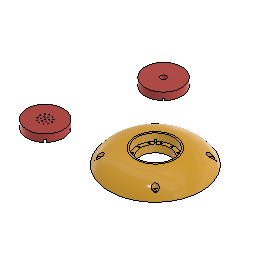
Chapeau (Autodesk Fusion 360 design; units mm, degrees)
Autodesk Fusion 360 part; units mm, degrees
note: some values were not read from the file. Set by a fixed rule: which sketch regions a step uses.
sketch "Sketch1" plane through (0, 0, 0) normal (0, 0, 1) x (1, 0, 0) in component "Chapeau"
  line L0 (-67.3, 67.3) -> (-82.7, 67.3)
  line L1 (-82.7, 67.3) -> (-82.7, 82.7)
  line L2 (-82.7, 82.7) -> (-67.3, 82.7)
  line L3 (-67.3, 82.7) -> (-67.3, 67.3)
  line L4 (-67.3, 67.3) -> (-82.7, 82.7) construction
  line L5 (-82.7, 67.3) -> (-67.3, 82.7) construction
  line L6 (0, 0) -> (0, 45.9001) construction
  line L7 (0, 0) -> (-36.9547, 0) construction
  line L8 (67.3, 82.7) -> (82.7, 82.7)
  line L9 (82.7, 82.7) -> (82.7, 67.3)
  line L10 (82.7, 67.3) -> (67.3, 67.3)
  line L11 (67.3, 67.3) -> (67.3, 82.7)
  line L12 (-82.7, -67.3) -> (-67.3, -67.3)
  line L13 (-67.3, -67.3) -> (-67.3, -82.7)
  line L14 (-67.3, -82.7) -> (-82.7, -82.7)
  line L15 (-82.7, -82.7) -> (-82.7, -67.3)
  line L16 (67.3, -67.3) -> (82.7, -67.3)
  line L17 (82.7, -67.3) -> (82.7, -82.7)
  line L18 (82.7, -82.7) -> (67.3, -82.7)
  line L19 (67.3, -82.7) -> (67.3, -67.3)
  circle A0 centre (0, 0) radius 125
  circle A1 centre (-75, 75) radius 3.1
  circle A2 centre (75, 75) radius 3.1
  circle A3 centre (-75, -75) radius 3.1
  circle A4 centre (75, -75) radius 3.1
  point P0 (-75, 75)
  dimension "d1" = 15.4
  dimension "d2" = 15.4
  dimension "d3" = 75
  dimension "d4" = 75
  dimension "d7" = 150
  dimension "d8" = -150
  dimension "d9" = 250
  dimension "d16" = 6.2
  dimension "d19" = 150
  dimension "d20" = -150
  constraint horizontal L0
  constraint perpendicular L0 L1
  constraint parallel L0 L2
  constraint parallel L1 L3
  constraint coincident L4 P0
  constraint coincident L5 P0
  constraint coincident L6.start L7.start
  constraint perpendicular L2 L6
  constraint perpendicular L6 L7
  constraint coincident P0 A1.centre
  measures "d1" distance of L1.end L2.end
  measures "d2" distance of L0.end L1.end
  measures "d3" vertical distance of L6.start A1.centre
  measures "d4" horizontal distance of L6.start A1.centre
  measures "d9" diameter of A0
  measures "d16" diameter of A1
extrude "Extrude1" add sketch "Sketch1" along normal blind 40 contours L0 L1 L2 L3 | L8 L9 L10 L11 | L12 L13 L14 L15 | L16 L17 L18 L19 | A0 | A1 | A2 | A3 | A4 makes body 1 in component "Chapeau"
fillet "Fillet1" radius 82.5 1 edges at (-116.5409, -45.2019, 40) on bodies 1 in component "Chapeau"
extrude "Extrude3" cut sketch "Sketch1" along normal blind 60 contours A1 | A2 | A3 | A4 bodies 1 in component "Chapeau"
extrude "Extrude2" cut sketch "Sketch1" along normal blind 10 contours L0 L1 L2 L3 | L8 L9 L10 L11 | L12 L13 L14 L15 | L16 L17 L18 L19 | A1 | A2 | A3 | A4 bodies 1 in component "Chapeau"
ref_plane "WorkPlane1" through (-75, 75, 14) normal (0, 0, -1) x (-1, 0, 0) in component "Chapeau"
sketch "Sketch2" plane through (75, -75, 14) normal (0, 0, -1) x (1, 0, 0) in component "Chapeau"
  circle A0 centre (-150, 0) radius 3.1
  circle A1 centre (-150, -150) radius 3.1
  circle A2 centre (0, -150) radius 3.1
  circle A3 centre (0, 0) radius 3.1
  circle A4 centre (-150, 0) radius 7.5
  circle A5 centre (-150, -150) radius 7.5
  circle A6 centre (0, -150) radius 7.5
  circle A7 centre (0, 0) radius 7.5
  dimension "d34" = 15
  dimension "d35" = 15
  dimension "d36" = 15
  dimension "d37" = 15
  constraint concentric A0 A4
  constraint concentric A1 A5
  constraint concentric A2 A6
  constraint concentric A3 A7
  measures "d34" diameter of A4
  measures "d35" diameter of A5
  measures "d36" diameter of A6
  measures "d37" diameter of A7
extrude "Extrude1'" cut sketch "Sketch2" against normal blind 55 bodies 1 in component "Chapeau"
sketch "Sketch4" plane through (0, 0, 40) normal (0, 0, 1) x (-1, 0, 0) in component "Chapeau"
  circle A0 centre (0, 0) radius 54.2893
  circle A1 centre (0, 0) radius 50
  circle A2 centre (0, 0) radius 40
  dimension "d53" = 100
  dimension "d54" = 10
  constraint concentric A0 A1
  constraint concentric A1 A2
  measures "d53" diameter of A1
  measures "d54" distance of A1 A2
extrude "Extrude3'" cut sketch "Sketch4" against normal through all contours A2 bodies 1 in component "Chapeau"
extrude "Extrude7" cut sketch "Sketch4" against normal blind 20 contours A1 bodies 1 in component "Chapeau"
sketch "Sketch1 (1)" plane through (0, 0, 20) normal (0, 0, 1) x (-1, 0, 0) in component "Chapeau"
  circle A0 centre (0, 0) radius 40
  circle A1 centre (0, 0) radius 54.2893
  circle A2 centre (0, -45) radius 2.5
  circle A3 centre (38.9711, -22.5) radius 2.5
  circle A4 centre (38.9711, 22.5) radius 2.5
  circle A5 centre (0, 45) radius 2.5
  circle A6 centre (-38.9711, 22.5) radius 2.5
  circle A7 centre (-38.9711, -22.5) radius 2.5
  circle A8 centre (0, -45) radius 1
  circle A9 centre (38.9711, -22.5) radius 1
  circle A10 centre (38.9711, 22.5) radius 1
  circle A11 centre (0, 45) radius 1
  circle A12 centre (-38.9711, 22.5) radius 1
  circle A13 centre (-38.9711, -22.5) radius 1
  circle A14 centre (0, 0) radius 40
  circle A15 centre (0, 0) radius 50
  line L0 (0, 0) -> (0, -40) construction
  line L1 (0, -40) -> (0, -50) construction
  line L2 (0, 0) -> (-40, 0) construction
  line L3 (-40, 0) -> (-50, 0) construction
  circle A16 centre (-45, 0) radius 2.1
  circle A17 centre (-22.5, -38.9711) radius 2.1
  circle A18 centre (22.5, -38.9711) radius 2.1
  circle A19 centre (45, 0) radius 2.1
  circle A20 centre (22.5, 38.9711) radius 2.1
  circle A21 centre (-22.5, 38.9711) radius 2.1
  line L4 (35.3553, -35.3553) -> (-35.3553, 35.3553) construction
  line L5 (37.0789, -33.5434) -> (-33.5434, 37.0789)
  line L6 (33.5434, -37.0789) -> (-37.0789, 33.5434)
  dimension "d58" = 5
  dimension "d60" = 360
  dimension "d61" = 2
  dimension "d72" = 4.2
  dimension "d74" = 360
  dimension "d76" = 45
  dimension "d77" = 2.5
  dimension "d78" = 2.5
  constraint concentric A2 A8
  constraint coincident A0.centre A1.centre
  constraint coincident A14 L0.end
  constraint vertical L0
  constraint coincident A15 L1.end
  constraint parallel L0 L1
  constraint midpoint A2.centre L1
  constraint coincident A14 L2.end
  constraint perpendicular L0 L2
  constraint coincident A15 L3.end
  constraint parallel L2 L3
  constraint midpoint L3 A16.centre
  constraint coincident A15 L4.start
  constraint coincident A15 L4.end
  constraint coincident A0.centre L4
  constraint coincident A15 L5.start
  constraint coincident A15 L5.end
  constraint coincident A15 L6.start
  constraint coincident A15 L6.end
  constraint parallel L4 L6
  constraint parallel L4 L5
  measures "d58" diameter of A2
  measures "d61" diameter of A8
  measures "d72" diameter of A16
  measures "d76" angle of L0 L4
  measures "d77" distance of L4 L5
  measures "d78" distance of L4 L6
extrude "Extrude5" cut sketch "Sketch1 (1)" against normal blind 4 contours A8 | A9 | A10 | A11 | A12 | A13 bodies 1 in component "Chapeau"
extrude "Extrude6" cut sketch "Sketch1 (1)" against normal blind 3 contours A2 | A3 | A4 | A5 | A6 | A7 bodies 1 in component "Chapeau"
extrude "Extrude8" cut sketch "Sketch1 (1)" against normal through all contours A16 | A17 | A18 | A19 | A20 | A21 bodies 1 in component "Chapeau"
extrude "Extrude9" add sketch "Sketch1 (1)" along normal blind 5 contours A0 A14 A15 L5 L6 | A0 A14 A15 L5 L6 bodies 1 in component "Chapeau"
sketch "Sketch2 (2)" plane through (0, 0, 0) normal (0, 0, 1) x (1, 0, 0) in component "Couvercle_1"
  circle A0 centre (0, 0) radius 49.5
  circle A1 centre (0, 45) radius 1
  circle A2 centre (38.9711, -22.5) radius 1
  circle A3 centre (38.9711, 22.5) radius 2.5
  circle A4 centre (-45, 0) radius 2.1
  line L0 (36.7919, -33.115) -> (-33.115, 36.7919)
  line L1 (0, 0) -> (-40, 0) construction
  circle A5 centre (-22.5, 38.9711) radius 2.1
  circle A6 centre (38.9711, -22.5) radius 2.5
  circle A7 centre (22.5, -38.9711) radius 2.1
  circle A8 centre (0, 45) radius 2.5
  line L2 (0, 0) -> (0, -40) construction
  circle A9 centre (38.9711, 22.5) radius 1
  circle A10 centre (-22.5, -38.9711) radius 2.1
  circle A11 centre (-38.9711, 22.5) radius 2.5
  circle A12 centre (45, 0) radius 2.1
  circle A13 centre (0, -45) radius 2.5
  circle A14 centre (-38.9711, -22.5) radius 1
  circle A15 centre (-38.9711, -22.5) radius 2.5
  line L3 (33.115, -36.7919) -> (-36.7919, 33.115)
  circle A16 centre (0, -45) radius 1
  circle A17 centre (22.5, 38.9711) radius 2.1
  line L4 (35.0018, -35.0018) -> (-35.0018, 35.0018) construction
  circle A18 centre (-38.9711, 22.5) radius 1
  circle A19 centre (0, 0) radius 40
  line L5 (0, -40) -> (0, -45) construction
  line L6 (-45, 0) -> (-40, 0) construction
  line L7 (-25.3851, 29.0621) -> (-29.0621, 25.3851)
  line L8 (25.3851, -29.0621) -> (29.0621, -25.3851)
  dimension "d82" = 360
  dimension "d84" = 360
  dimension "d85" = 5
  dimension "d86" = 2
  dimension "d87" = 4.2
  dimension "d88" = 45
  dimension "d89" = 2.6
  dimension "d90" = 2.6
  dimension "d91" = 99
  dimension "d92" = 80
  dimension "d93" = 45
  dimension "d94" = 45
  dimension "d103" = 11
  dimension "d104" = 11
  constraint concentric A13 A16
  constraint coincident A0.centre L1.start
  constraint coincident L2.end A19
  constraint vertical L2
  constraint coincident L1.end A19
  constraint perpendicular L1 L2
  constraint coincident L4.start A0
  constraint coincident L4.end A0
  constraint coincident A0.centre L4
  constraint coincident L0.start A0
  constraint coincident L0.end A0
  constraint coincident L3.start A0
  constraint coincident L3.end A0
  constraint parallel L3 L4
  constraint parallel L0 L4
  constraint coincident A13.centre A16.centre
  constraint parallel L2 L5
  constraint coincident A4.centre L6.start
  constraint parallel L1 L6
  constraint coincident L0 L7.start
  constraint coincident L3 L7.end
  constraint perpendicular L3 L7
  constraint coincident L3 L8.start
  constraint coincident L0 L8.end
  constraint perpendicular L0 L8
  measures "d85" diameter of A13
  measures "d86" diameter of A16
  measures "d87" diameter of A4
  measures "d88" angle of L2 L4
  measures "d89" distance of L0 L4
  measures "d90" distance of L3 L4
  measures "d91" diameter of A0
  measures "d92" diameter of A19
  measures "d93" distance of A13.centre A0.centre
  measures "d94" distance of A0.centre A4.centre
  measures "d103" distance of L4.end L7
  measures "d104" distance of L4.start L8
extrude "Extrude1''" add sketch "Sketch2 (2)" along normal blind 20 separate body contours A0 L0 A19 | A0 L0 L3 A19 | A0 L0 L3 A19 | A0 L3 A19 | L0 A19 | L0 L3 A19 L7 | L0 L3 A19 L8 | L3 A19 | L0 L3 L7 L8 | A1 | A2 | A3 | A4 | A5 | A6 | A7 | A8 | A9 | A10 | A11 | A12 | A13 | A14 | A15 | A16 | A17 | A18 makes body 2 in component "Couvercle_1"
extrude "Extrude2'" cut sketch "Sketch2 (2)" along normal blind 4 contours A1 | A2 | A9 | A14 | A16 | A18 bodies 2 in component "Couvercle_1"
extrude "Extrude3''" cut sketch "Sketch2 (2)" along normal blind 3.2 contours A3 | A6 | A8 | A11 | A13 | A15 bodies 2 in component "Couvercle_1"
extrude "Extrude4" cut sketch "Sketch2 (2)" along normal blind 6 contours A0 L0 L3 A19 | A0 L0 L3 A19 | L0 L3 A19 L7 | L0 L3 A19 L8 bodies 2 in component "Couvercle_1"
sketch "Sketch2 (3)" plane through (0, 0, 0) normal (0, 0, 1) x (1, 0, 0) in component "Couvercle_2"
  circle A0 centre (0, 0) radius 49.5
  circle A1 centre (0, 45) radius 1
  circle A2 centre (38.9711, -22.5) radius 1
  circle A3 centre (38.9711, 22.5) radius 2.5
  circle A4 centre (-45, 0) radius 2.1
  line L0 (36.7919, -33.115) -> (-33.115, 36.7919)
  line L1 (0, 0) -> (-40, 0) construction
  circle A5 centre (-22.5, 38.9711) radius 2.1
  circle A6 centre (38.9711, -22.5) radius 2.5
  circle A7 centre (22.5, -38.9711) radius 2.1
  circle A8 centre (0, 45) radius 2.5
  line L2 (0, 0) -> (0, -40) construction
  circle A9 centre (38.9711, 22.5) radius 1
  circle A10 centre (-22.5, -38.9711) radius 2.1
  circle A11 centre (-38.9711, 22.5) radius 2.5
  circle A12 centre (45, 0) radius 2.1
  circle A13 centre (0, -45) radius 2.5
  circle A14 centre (-38.9711, -22.5) radius 1
  circle A15 centre (-38.9711, -22.5) radius 2.5
  line L3 (33.115, -36.7919) -> (-36.7919, 33.115)
  circle A16 centre (0, -45) radius 1
  circle A17 centre (22.5, 38.9711) radius 2.1
  line L4 (35.0018, -35.0018) -> (-35.0018, 35.0018) construction
  circle A18 centre (-38.9711, 22.5) radius 1
  circle A19 centre (0, 0) radius 40
  line L5 (0, -40) -> (0, -45) construction
  line L6 (-45, 0) -> (-40, 0) construction
  line L7 (-25.3851, 29.0621) -> (-29.0621, 25.3851)
  line L8 (25.3851, -29.0621) -> (29.0621, -25.3851)
  dimension "d82_1" = 360
  dimension "d84_1" = 360
  dimension "d85_1" = 5
  dimension "d86_1" = 2
  dimension "d87_1" = 4.2
  dimension "d88_1" = 45
  dimension "d89_1" = 2.6
  dimension "d90_1" = 2.6
  dimension "d91_1" = 99
  dimension "d92_1" = 80
  dimension "d93_1" = 45
  dimension "d94_1" = 45
  dimension "d103_1" = 11
  dimension "d104_1" = 11
  constraint concentric A13 A16
  constraint coincident A0.centre L1.start
  constraint coincident L2.end A19
  constraint vertical L2
  constraint coincident L1.end A19
  constraint perpendicular L1 L2
  constraint coincident L4.start A0
  constraint coincident L4.end A0
  constraint coincident A0.centre L4
  constraint coincident L0.start A0
  constraint coincident L0.end A0
  constraint coincident L3.start A0
  constraint coincident L3.end A0
  constraint parallel L3 L4
  constraint parallel L0 L4
  constraint coincident A13.centre A16.centre
  constraint parallel L2 L5
  constraint coincident A4.centre L6.start
  constraint parallel L1 L6
  constraint coincident L0 L7.start
  constraint coincident L3 L7.end
  constraint perpendicular L3 L7
  constraint coincident L3 L8.start
  constraint coincident L0 L8.end
  constraint perpendicular L0 L8
  measures "d85_1" diameter of A13
  measures "d86_1" diameter of A16
  measures "d87_1" diameter of A4
  measures "d88_1" angle of L2 L4
  measures "d89_1" distance of L0 L4
  measures "d90_1" distance of L3 L4
  measures "d91_1" diameter of A0
  measures "d92_1" diameter of A19
  measures "d93_1" distance of A13.centre A0.centre
  measures "d94_1" distance of A0.centre A4.centre
  measures "d103_1" distance of L4.end L7
  measures "d104_1" distance of L4.start L8
extrude "Extrude1'''" add sketch "Sketch2 (3)" along normal blind 20 separate body contours A0 L0 A19 | A0 L0 L3 A19 | A0 L0 L3 A19 | A0 L3 A19 | L0 A19 | L0 L3 A19 L7 | L0 L3 A19 L8 | L3 A19 | L0 L3 L7 L8 | A1 | A2 | A3 | A4 | A5 | A6 | A7 | A8 | A9 | A10 | A11 | A12 | A13 | A14 | A15 | A16 | A17 | A18 makes body 3 in component "Couvercle_2"
extrude "Extrude2''" cut sketch "Sketch2 (3)" along normal blind 4 contours A1 | A2 | A9 | A14 | A16 | A18 bodies 3 in component "Couvercle_2"
extrude "Extrude3'''" cut sketch "Sketch2 (3)" along normal blind 3.2 contours A3 | A6 | A8 | A11 | A13 | A15 bodies 3 in component "Couvercle_2"
extrude "Extrude4'" cut sketch "Sketch2 (3)" along normal blind 6 contours A0 L0 L3 A19 | A0 L0 L3 A19 | L0 L3 A19 L7 | L0 L3 A19 L8 bodies 3 in component "Couvercle_2"
sketch "Sketch4 (2)" plane through (0, 0, 20) normal (0, 0, 1) x (-1, 0, 0) in component "Couvercle_2"
  circle A0 centre (0, 0) radius 49.5
  circle A1 centre (0, 0) radius 1.25
  circle A2 centre (0, 0) radius 2.5
  circle A3 centre (0, 8) radius 1.25
  circle A4 centre (0, 8) radius 2.5
  circle A5 centre (0, 16) radius 1.25
  circle A6 centre (0, 16) radius 2.5
  circle A7 centre (-6.9282, 4) radius 2.5
  circle A8 centre (-6.9282, 4) radius 1.25
  circle A9 centre (-6.9282, -4) radius 2.5
  circle A10 centre (-6.9282, -4) radius 1.25
  circle A11 centre (0, -8) radius 2.5
  circle A12 centre (0, -8) radius 1.25
  circle A13 centre (6.9282, -4) radius 2.5
  circle A14 centre (6.9282, -4) radius 1.25
  circle A15 centre (6.9282, 4) radius 2.5
  circle A16 centre (6.9282, 4) radius 1.25
  circle A17 centre (-8.6503, 13.4601) radius 2.5
  circle A18 centre (-8.6503, 13.4601) radius 1.25
  circle A19 centre (-14.5541, 6.6466) radius 2.5
  circle A20 centre (-14.5541, 6.6466) radius 1.25
  circle A21 centre (-15.8371, -2.277) radius 2.5
  circle A22 centre (-15.8371, -2.277) radius 1.25
  circle A23 centre (-12.092, -10.4778) radius 2.5
  circle A24 centre (-12.092, -10.4778) radius 1.25
  circle A25 centre (-4.5077, -15.3519) radius 2.5
  circle A26 centre (-4.5077, -15.3519) radius 1.25
  circle A27 centre (4.5077, -15.3519) radius 2.5
  circle A28 centre (4.5077, -15.3519) radius 1.25
  circle A29 centre (12.092, -10.4778) radius 2.5
  circle A30 centre (12.092, -10.4778) radius 1.25
  circle A31 centre (15.8371, -2.277) radius 2.5
  circle A32 centre (15.8371, -2.277) radius 1.25
  circle A33 centre (14.5541, 6.6466) radius 2.5
  circle A34 centre (14.5541, 6.6466) radius 1.25
  circle A35 centre (8.6503, 13.4601) radius 2.5
  circle A36 centre (8.6503, 13.4601) radius 1.25
  dimension "d110" = 2.5
  dimension "d111" = 5
  dimension "d117" = 0
  dimension "d118" = 8
  dimension "d120" = 360
  dimension "d122" = 360
  constraint concentric A1 A2
  constraint coincident A0.centre A1.centre
  measures "d110" diameter of A1
  measures "d111" diameter of A2
extrude "Extrude5'" cut sketch "Sketch4 (2)" against normal through all contours A1 | A3 | A5 | A8 | A10 | A12 | A14 | A16 | A18 | A20 | A22 | A24 | A26 | A28 | A30 | A32 | A34 | A36 bodies 3 in component "Couvercle_2"
extrude "Extrude6'" cut sketch "Sketch4 (2)" against normal through all from surface at -10 contours A2 | A4 | A6 | A7 | A9 | A11 | A13 | A15 | A17 | A19 | A21 | A23 | A25 | A27 | A29 | A31 | A33 | A35 bodies 3 in component "Couvercle_2"
sketch "Sketch5" plane through (0, 0, 124.3049) normal (0, 0, 1) x (-1, 0, 0)
  circle A0 centre (50.9471, -73.3578) radius 49.5
  circle A1 centre (50.9471, -73.3578) radius 7.5
  line L0 (76.3322, -102.4199) -> (84.0621, -110.1497)
  arc A2 (14.1552, -40.2428) -> (84.0621, -110.1497) centre (50.9471, -73.3578) ccw
  line L1 (14.1552, -40.2428) -> (21.885, -47.9726)
  line L2 (21.885, -47.9726) -> (25.562, -44.2957)
  line L3 (25.562, -44.2957) -> (17.8321, -36.5658)
  arc A3 (87.7391, -106.4728) -> (17.8321, -36.5658) centre (50.9471, -73.3578) ccw
  line L4 (87.7391, -106.4728) -> (80.0092, -98.7429)
  line L5 (80.0092, -98.7429) -> (76.3322, -102.4199)
  circle A4 centre (11.976, -95.8578) radius 2.5
  circle A5 centre (89.9183, -50.8578) radius 2.5
  circle A6 centre (50.9471, -118.3578) radius 2.5
  circle A7 centre (11.976, -50.8578) radius 2.5
  circle A8 centre (50.9471, -28.3578) radius 2.5
  circle A9 centre (89.9183, -95.8578) radius 2.5
  circle A10 centre (50.9471, -73.3578) radius 7
  circle A11 centre (50.9471, -73.3578) radius 9
  dimension "d126" = 15
  dimension "d129" = 14
  dimension "d130" = 18
  constraint concentric A0 A1
  constraint concentric A0 A10
  constraint concentric A10 A11
  measures "d126" diameter of A1
  measures "d129" diameter of A10
  measures "d130" diameter of A11
extrude "Extrude5''" cut sketch "Sketch5" along normal up to surface (20 mm away) contours A1 | A10 sketch seen with x (1, 0, 0) y (0, 1, 0) z (0, 0, 1) at (50.9471, -73.3578, -124.3049) bodies 2 in component "Couvercle_1"
extrude "Extrude6''" add sketch "Sketch5" against normal blind 1 contours A1 | A11 sketch seen with x (1, 0, 0) y (0, 1, 0) z (0, 0, 1) at (50.9471, -73.3578, -124.3049) bodies 2 in component "Couvercle_1"
fillet "Fillet1'" radius 5 1 edges at (8.3909, 3.2545, 0) on bodies 2 in component "Couvercle_1"
fillet "Fillet2" radius 0.5 1 edges at (6.5263, -2.5313, 0) on bodies 2 in component "Couvercle_1"
component "Chapeau" placed x (1, 0, 0) y (0, 1, 0) z (0, 0, 1) at (0, 0, 0)
component "Couvercle_1" placed x (1, 0, 0) y (0, 1, 0) z (0, 0, 1) at (-50.9471, 73.3578, 124.3049)
component "Couvercle_2" placed x (1, 0, 0) y (0, 1, 0) z (0, 0, 1) at (-179.0991, -120.6434, 58.4556)
equation "Diam_trou = 4.2 mm"
equation "d72 = Diam_trou"
equation "d87 = Diam_trou"
equation "d87_1 = Diam_trou"
named bodies: "Chapeau Mignon", "Couvercle Mignon"
